Autodesk Inventor part; units mm, degrees
(part 2 of 2)
sketch "Esboço53" plane through (0, 44, 0) normal (0, 1, 0) x (1, 0, 0)
  point P0 (0, 0)
extrude "Extrusão37" add sketch "Esboço49" against normal blind 44 contours A1 L5 L6 L1 L0 | L2 L3 L9 A0 | L10 L12 L13 A2 | L11 L19 A3 L16 L17 L21 L20 | A2 L11 L14 L15 | L22 L24 A4 L26 | L24 L25 A4
sketch "Esboço54" plane through (0, 44, 0) normal (0, 1, 0) x (1, 0, 0)
  line L0 (-10, 63.5) -> (-10, 66.5) projected
  circle A0 centre (-10, 65) radius 1.5
  point P0 (0, 0)
  constraints: 1 centre point, 1 midpoint
extrude "Extrusão38" cut sketch "Esboço54" against normal blind 10
thread "Rosca13" size "M3x0.5" class "6H" standard "ANSI Metric M Profile" length 11
sketch "Esboço55" plane through (0, 16, 0) normal (0, 1, 0) x (1, 0, 0)
  line L0 (-41, 51.5) -> (-62.5, 51.5) projected
  line L1 (-65, 43.5) -> (-41, 43.5) projected
  line L2 (-62.5, 51.5) -> (-65, 51.5)
  line L3 (-65, 51.5) -> (-65, 43.5)
  line L4 (-65, 43.5) -> (-62.5, 43.5)
  line L5 (-62.5, 43.5) -> (-62.5, 51.5)
  line L6 (-62.5, 23.5) -> (-41, 23.5) projected
  line L7 (-41, 31.5) -> (-65, 31.5) projected
  line L8 (-62.5, 23.5) -> (-65, 23.5)
  line L9 (-65, 23.5) -> (-65, 31.5)
  line L10 (-65, 31.5) -> (-62.5, 31.5)
  line L11 (-62.5, 31.5) -> (-62.5, 23.5)
  line L12 (-10, 51.5) -> (-10, 23.5) projected
  line L13 (-10, 51.5) -> (-12.5, 51.5)
  line L14 (-12.5, 51.5) -> (-12.5, 43.5)
  line L15 (-12.5, 43.5) -> (-10, 43.5)
  line L16 (-10, 43.5) -> (-10, 51.5)
  line L17 (-10, 31.5) -> (-12.5, 31.5)
  line L18 (-12.5, 31.5) -> (-12.5, 23.5)
  line L19 (-12.5, 23.5) -> (-10, 23.5)
  line L20 (-10, 23.5) -> (-10, 31.5)
  point P0 (0, 0)
  constraints: 32 end point, 8 parallel, 5 point on line, 4 horizontal, 4 perpendicular
extrude "Extrusão39" add sketch "Esboço55" along normal blind 28
sketch "Esboço56" plane through (0, 44, 0) normal (0, 1, 0) x (1, 0, 0)
  point P0 (0, 0)
sketch "Esboço58" plane through (0, 44, 0) normal (0, 1, 0) x (1, 0, 0)
  line L0 (-34, 31.5) -> (-10, 31.5) projected
  line L1 (-34, 43.5) -> (-12.5, 43.5) projected
  line L2 (-10, 43.5) -> (-10, 31.5) projected
  line L3 (-12.5, 43.5) -> (-10, 43.5)
  line L4 (-10, 43.5) -> (-10, 31.5)
  line L5 (-10, 31.5) -> (-12.5, 31.5)
  line L6 (-12.5, 31.5) -> (-12.5, 43.5)
  line L7 (-65, 31.5) -> (-65, 43.5) projected
  line L8 (-62.5, 65) -> (-62.5, 10) projected
  line L9 (-65, 43.5) -> (-62.5, 43.5)
  line L10 (-62.5, 43.5) -> (-62.5, 31.5)
  line L11 (-62.5, 31.5) -> (-65, 31.5)
  line L12 (-65, 31.5) -> (-65, 43.5)
  line L13 (-5, 31.5) -> (-3, 31.5)
  line L14 (-3, 31.5) -> (-3, 20)
  line L15 (-3, 20) -> (-5, 20)
  line L16 (-12.5, 31.5) -> (-34, 31.5) projected
  line L17 (-12.5, 31.5) -> (-12.5, 29)
  line L18 (-12.5, 23.5) -> (-12.5, 31.5) projected
  line L19 (-5, 70) -> (-5, 5) projected
  line L20 (-12.5, 29) -> (-5, 29)
  line L21 (-5, 29) -> (-5, 5)
  line L22 (-5, 5) -> (-12.5, 5)
  line L23 (-12.5, 5) -> (-12.5, 29)
  point P0 (0, 0)
  point P1 (-12.4975, 31.5)
  constraints: 32 end point, 7 parallel, 4 horizontal, 4 perpendicular, 4 point on line
extrude "Extrusão40" add sketch "Esboço58" against normal blind 5 contours L6 L3 L2 L0 | L7 L9 L8 L11
extrude "Extrusão42" cut sketch "Esboço58" against normal blind 2 contours L20 L19 L22 L23 L18
sketch "Esboço59" plane through (0, 64, 0) normal (0, 1, 0) x (1, 0, 0)
  line L0 (-5, 5) -> (-10, 5)
  line L1 (-10, 5) -> (-10, 2)
  line L2 (-10, 2) -> (-5, 2)
  line L3 (-5, 2) -> (-5, 5)
  point P0 (0, 0)
  constraints: 8 end point, 2 parallel, 1 horizontal, 1 perpendicular
extrude "Extrusão43" cut sketch "Esboço59" against normal blind 22
sketch "Esboço60" plane through (0, 44, 0) normal (0, 1, 0) x (1, 0, 0)
  line L0 (-62.5, 51.5) -> (-62.5, 43.5) projected
  line L1 (-62.5, 51.5) -> (-62.5, 54)
  line L2 (-62.5, 67) -> (-62.5, 51.5) projected
  line L3 (-70, 70) -> (-70, 5) projected
  line L4 (-62.5, 54) -> (-70, 54)
  line L5 (-70, 54) -> (-70, 70)
  line L6 (-70, 70) -> (-62.5, 70)
  line L7 (-62.5, 70) -> (-62.5, 54)
  point P0 (0, 0)
  constraints: 10 end point, 2 parallel, 1 horizontal, 1 perpendicular, 1 point on line
sketch "Esboço61" plane through (0, 64, 0) normal (0, 1, 0) x (1, 0, 0)
  line L0 (-70, 70) -> (-55.5, 70) projected
  line L1 (-70, 70) -> (-65, 70)
  line L2 (-65, 70) -> (-65, 73)
  line L3 (-65, 73) -> (-70, 73)
  line L4 (-70, 73) -> (-70, 70)
  point P0 (0, 0)
  constraints: 8 end point, 2 parallel, 1 horizontal, 1 perpendicular
extrude "Extrusão44" cut sketch "Esboço60" against normal blind 2
extrude "Extrusão45" cut sketch "Esboço61" against normal blind 22
sketch "Esboço62" plane through (0, 0, 0) normal (0, -1, 0) x (1, 0, 0)
  line L0 (-8, -54.8494) -> (-8, -20.1506) projected
  line L1 (-8, -54.8494) -> (-67, -54.8494)
  line L2 (-67, -54.8494) -> (-67, -20.1506)
  line L3 (-67, -20.1506) -> (-8, -20.1506)
  line L4 (-8, -20.1506) -> (-8, -54.8494)
  point P0 (0, 0)
  constraints: 8 end point, 2 parallel, 1 horizontal, 1 perpendicular
extrude "Extrusão46" cut sketch "Esboço62" against normal blind 2
sketch "Esboço65" plane through (0, 44, 0) normal (0, 1, 0) x (1, 0, 0)
  line L0 (-5, 29) -> (-5, 31.5)
  point P0 (0, 0)
  constraints: 2 end point
sketch "Esboço68" plane through (0, 44, 0) normal (0, 1, 0) x (1, 0, 0)
  line L0 (-62.5, 43.5) -> (-62.5, 31.5) projected
  line L1 (-62.5, 43.5) -> (-62.5, 46)
  line L2 (-62.5, 51.5) -> (-62.5, 43.5) projected
  line L3 (-70, 54) -> (-70, 5) projected
  line L4 (-70, 54) -> (-62.5, 54)
  line L5 (-62.5, 54) -> (-62.5, 46)
  line L6 (-62.5, 46) -> (-70, 46)
  line L7 (-70, 46) -> (-70, 54)
  point P0 (0, 0)
  constraints: 10 end point, 2 parallel, 1 horizontal, 1 perpendicular, 1 point on line
extrude "Extrusão47" cut sketch "Esboço68" against normal blind 2
sketch "Esboço69" plane through (0, 64, 0) normal (0, 1, 0) x (1, 0, 0)
  point P0 (0, 0)
sketch "Esboço70" plane through (0, 16, 0) normal (0, 1, 0) x (1, 0, 0)
  line L0 (-41, 43.5) -> (-41, 51.5) projected
  line L1 (-41, 31.5) -> (-34, 31.5) projected
  line L2 (-41, 43.5) -> (-39.1, 43.5)
  line L3 (-39.1, 43.5) -> (-39.1, 31.5)
  line L4 (-39.1, 31.5) -> (-41, 31.5)
  line L5 (-41, 31.5) -> (-41, 43.5)
  line L6 (-34, 31.5) -> (-34, 43.5) projected
  line L7 (-34, 43.5) -> (-35.9, 43.5)
  line L8 (-35.9, 43.5) -> (-35.9, 31.5)
  line L9 (-35.9, 31.5) -> (-34, 31.5)
  line L10 (-34, 31.5) -> (-34, 43.5)
  point P0 (0, 0)
  dimension "d227" = 1.9
  dimension "d228" = 1.9
  constraints: 16 end point, 4 parallel, 2 horizontal, 2 perpendicular, 2 point on line
  measures "d227" distance of L3.end L4.end
  measures "d228" distance of L9.end L8.end
extrude "Extrusão48" cut sketch "Esboço70" against normal blind 4
sketch "Esboço71" plane through (0, 16, 0) normal (0, 1, 0) x (1, 0, 0)
  line L0 (-41, 43.5) -> (-41, 51.5) projected
  line L1 (-39.1, 43.5) -> (-39.1, 31.5) projected
  line L2 (-41, 51.5) -> (-39.1, 51.5)
  line L3 (-39.1, 51.5) -> (-39.1, 43.5)
  line L4 (-39.1, 43.5) -> (-41, 43.5)
  line L5 (-41, 43.5) -> (-41, 51.5)
  line L6 (-35.9, 43.5) -> (-34, 43.5) projected
  line L7 (-34, 51.5) -> (-35.9, 51.5)
  line L8 (-35.9, 51.5) -> (-35.9, 43.5)
  line L9 (-35.9, 43.5) -> (-34, 43.5)
  line L10 (-34, 43.5) -> (-34, 51.5)
  line L11 (-41, 23.5) -> (-41, 31.5) projected
  line L12 (-41, 23.5) -> (-39.1, 23.5)
  line L13 (-39.1, 23.5) -> (-39.1, 31.5)
  line L14 (-39.1, 31.5) -> (-41, 31.5)
  line L15 (-41, 31.5) -> (-41, 23.5)
  line L16 (-34, 31.5) -> (-34, 23.5) projected
  line L17 (-34, 23.5) -> (-35.9, 23.5)
  line L18 (-35.9, 23.5) -> (-35.9, 31.5)
  line L19 (-35.9, 31.5) -> (-34, 31.5)
  line L20 (-34, 31.5) -> (-34, 23.5)
  point P0 (0, 0)
  constraints: 32 end point, 8 parallel, 4 horizontal, 4 perpendicular, 4 point on line
extrude "Extrusão49" add sketch "Esboço71" against normal blind 14
